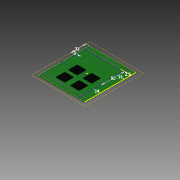
# Autodesk Inventor part: PCB
Saved by Autodesk Inventor 2015 SP1 (Build 190203100, 203)
## iProperties
Created: 2015-01-22
Part Number: PCB
Material: Generic
Document SubType Name: Modeling
Designer: Patrick
Density: 1 g/cm^3
Appearance: Default
Author: Patrick
Autodesk Inventor part; units mm, degrees
ref_plane "YZ Plane" through (0, 0, 0) normal (1, 0, 0) x (0, 1, 0)
ref_plane "XZ Plane" through (0, 0, 0) normal (0, 1, 0) x (-1, 0, 0)
ref_plane "XY Plane" through (0, 0, 0) normal (0, 0, 1) x (1, 0, 0)
sketch "Sketch1" plane through (0, 0, 0) normal (0, 0, 1) x (1, 0, 0)
  line L0 (-50, 55) -> (50, 55)
  line L1 (50, 55) -> (50, -55)
  line L2 (50, -55) -> (-50, -55)
  line L3 (-50, -55) -> (-50, 55)
  line L4 (-50, 55) -> (50, -55) construction
  line L5 (50, 55) -> (-50, -55) construction
  point P0 (0, 0)
  dimension "d0" = 100
  dimension "d1" = 110
  constraints: 12 end point, 2 midpoint, 2 parallel, 1 horizontal, 1 perpendicular
  measures "d0" distance of L1.end L2.end
  measures "d1" distance of L0.end L1.end
extrude "Extrusion1" add sketch "Sketch1" along normal blind 1.8
sketch "Sketch2" plane through (0, 0, 1.8) normal (0, 0, 1) x (1, 0, 0)
  line L0 (-26.5, -21.4) -> (-7.5, -21.4)
  line L1 (-7.5, -21.4) -> (-7.5, -40.4)
  line L2 (-7.5, -40.4) -> (-26.5, -40.4)
  line L3 (-26.5, -40.4) -> (-26.5, -21.4)
  line L4 (-26.5, -21.4) -> (-7.5, -40.4) construction
  line L5 (-7.5, -21.4) -> (-26.5, -40.4) construction
  line L6 (-50, -55) -> (50, -55) projected
  line L7 (-50, 55) -> (-50, -55) projected
  point P0 (0, 0)
  point P1 (-17, -30.9)
  dimension "d4" = 19
  dimension "d5" = 19
  dimension "d8" = 33.6
  dimension "d9" = 42.5
  constraints: 12 end point, 2 midpoint, 2 parallel, 1 horizontal, 1 perpendicular
  measures "d4" distance of L1.end L2.end
  measures "d5" distance of L0.end L1.end
  measures "d8" distance between parallel lines of L0 L6
  measures "d9" distance between parallel lines of L1 L7
extrude "Extrusion2" add sketch "Sketch2" along normal blind 1
pattern_linear "Rectangular Pattern1" count 2 spacing 31 along (1, 0, 0) count 2 spacing 27 along (0, 1, 0) of "Extrusion2"
sketch "Sketch3" plane through (0, 0, 1.8) normal (0, 0, 1) x (1, 0, 0)
  line L0 (-46.7, -46.1) -> (-26.7, -46.1) construction
  line L1 (-46.7, -47.2) -> (-26.7, -47.2)
  line L2 (-26.7, -45) -> (-46.7, -45)
  arc A0 (-46.7, -45) -> (-46.7, -47.2) centre (-46.7, -46.1) ccw
  arc A1 (-26.7, -47.2) -> (-26.7, -45) centre (-26.7, -46.1) ccw
  line L3 (-50, 55) -> (-50, -55) projected
  line L4 (-50, -55) -> (50, -55) projected
  point P0 (0, 0)
  point P1 (-36.7, -46.1)
  dimension "d16" = 20
  dimension "d17" = 2.2
  dimension "d18" = 2.2
  dimension "d19" = 7.8
  constraints: 8 end point, 4 point on circle, 4 tangent, 2 centre point, 1 horizontal, 1 midpoint, 1 parallel
  measures "d16" distance of L0.start L0.end
  measures "d17" diameter of A1
  measures "d18" distance edge to line of A0 L3
  measures "d19" distance between parallel lines of L4 L1
extrude "Extrusion3" cut sketch "Sketch3" against normal through all
pattern_linear "Rectangular Pattern2" count 4 spacing 24.6 along (1, 0, 0) count 2 spacing 92 along (0, 1, 0) of "Extrusion3"
sketch "Sketch4" plane through (0, 0, 1.8) normal (0, 0, 1) x (1, 0, 0)
  line L0 (50, -55) -> (50, 55) projected
  line L1 (50, 42.3) -> (-50.0933, 42.3) construction
  line L2 (47.1, 44.8) -> (27.1, 44.8) projected
  line L3 (50, -5.2) -> (-50.0933, -5.2) construction
  line L4 (35, 55) -> (35, -55) construction
  line L5 (36, 55) -> (36, -55) construction
  line L6 (-47, 55) -> (-47, -55) construction
  line L7 (-50, -55) -> (50, -55) construction
  line L8 (-50, 55) -> (-50, -55) construction
  line L9 (-50, 23) -> (-32.5921, 23) construction
  line L10 (50, 55) -> (-50, 55) construction
  line L11 (60.1599, 62.0026) -> (59.0568, -63.0375) construction
  line L12 (59.0568, -63.0375) -> (-57.4953, -62.0093) construction
  line L13 (-57.4953, -62.0093) -> (-56.3922, 63.0308) construction
  line L14 (-56.3922, 63.0308) -> (60.1599, 62.0026) construction
  point P0 (0, 0)
  dimension "d28" = 2.5
  dimension "d29" = 50
  dimension "d30" = 15
  dimension "d31" = 14
  dimension "d44" = 3
  dimension "d45" = 32
  constraints: 12 end point, 4 point on line, 3 vertical, 2 horizontal, 1 perpendicular, 2 other
  measures "d28" distance between parallel lines of L1 L2
  measures "d29" distance between parallel lines of L3 L2
  measures "d30" distance between parallel lines of L4 L0
  measures "d31" distance between parallel lines of L5 L0
  measures "d44" distance between parallel lines of L6 L8
  measures "d45" distance between parallel lines of L9 L10
sketch "Sketch5" plane through (0, 0, 1.8) normal (0, 0, 1) x (1, 0, 0)
  line L0 (-50, 55) -> (-50, -55) projected
  line L1 (50, -55) -> (50, 55) projected
  line L2 (50, 55) -> (-50, 55) projected
  line L3 (-50, -55) -> (50, -55) projected
  point P0 (0, 0)
  point P1 (-40, 51)
  point P2 (41, 51)
  point P3 (-40, -51)
  point P4 (40, -51)
  dimension "d32" = 10
  dimension "d33" = 9
  dimension "d34" = 4
  dimension "d36" = 4
  dimension "d88" = 10
  constraints: 2 horizontal alignment, 1 vertical alignment
  measures "d32" distance from line of L0 point (-40, 51)
  measures "d33" distance from line of L1 point (41, 51)
  measures "d34" distance from line of L2 point (41, 51)
  measures "d36" distance from line of L3 point (40, -51)
  measures "d88" distance from line of L1 point (40, -51)
hole "Hole1" at (-40, 51, 1.8) at (-40, -51, 1.8) at (40, -51, 1.8) at (41, 51, 1.8) direction (0, 0, -1) diameter 3 end through all
sketch "Sketch7" plane through (0, 0, 1.8) normal (0, 0, 1) x (1, 0, 0)
  point P0 (0, 0)
equation "\"d36\" = d34"
body "Solid1"
